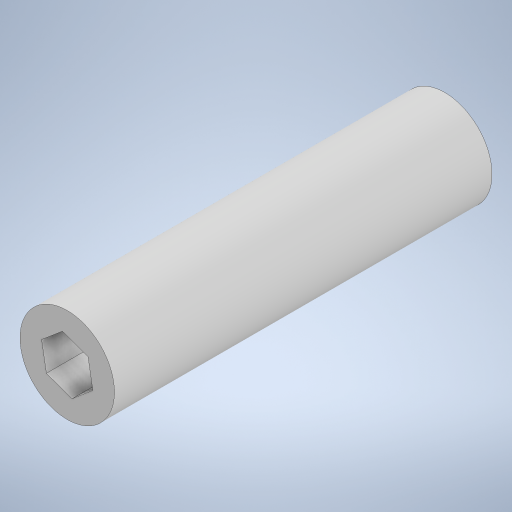
# Autodesk Inventor part: 4-bar intake mid roller
Saved by Autodesk Inventor 2023 (Build 270158030, 158C)
## iProperties
Created: 2022-07-19
Part Number: 4-bar intake mid roller
Material: Generic
Document SubType Name: Modeling
Designer: rm0990889
Density: 1 g/cm^3
Appearance: Default
Author: rm0990889
Autodesk Inventor part; units mm, degrees
ref_plane "YZ Plane" through (0, 0, 0) normal (1, 0, 0) x (0, 1, 0)
ref_plane "XZ Plane" through (0, 0, 0) normal (0, 1, 0) x (-1, 0, 0)
ref_plane "XY Plane" through (0, 0, 0) normal (0, 0, 1) x (1, 0, 0)
sketch "Sketch2" plane through (0, 0, 0) normal (0, 0, 1) x (1, 0, 0)
  circle A0 centre (0, 0) radius 12.7
  circle A1 centre (0, 0) radius 6.35
  line L0 (5.601, 4.732) -> (6.8985, -2.4846)
  line L1 (6.8985, -2.4846) -> (1.2975, -7.2166)
  line L2 (1.2975, -7.2166) -> (-5.601, -4.732)
  line L3 (-5.601, -4.732) -> (-6.8985, 2.4846)
  line L4 (-6.8985, 2.4846) -> (-1.2975, 7.2166)
  line L5 (-1.2975, 7.2166) -> (5.601, 4.732)
  point P0 (2.1518, 5.9743)
  dimension "d8" = 12.7
  dimension "d7" = 25.4
  constraints: 12 end point, 3 coincident, 1 centre point, 1 midpoint, 16 other
  measures "d7" diameter of A0
extrude "Extrusion1" add sketch "Sketch2" along normal blind 101.6
body "Solid1"
